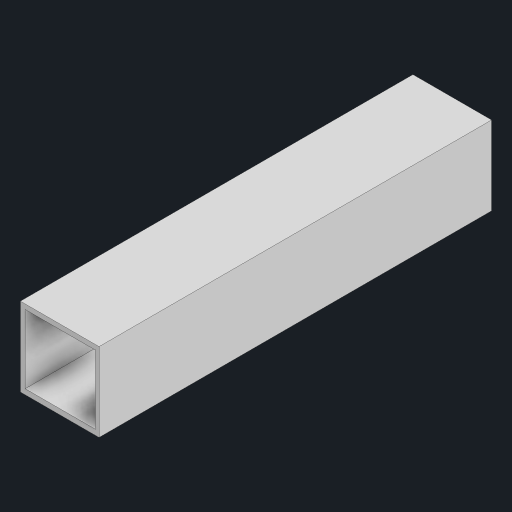
# Autodesk Inventor part: support
Saved by Autodesk Inventor 2024 (Build 280153000, 153)
## iProperties
Created: 2023-11-07
Part Number: support
Material: Generic
Document SubType Name: Modeling
Designer: 91840
Density: 1 g/cm^3
Appearance: Default
Author: 91840
Autodesk Inventor part; units mm, degrees
ref_plane "YZ Plane" through (0, 0, 0) normal (1, 0, 0) x (0, 1, 0)
ref_plane "XZ Plane" through (0, 0, 0) normal (0, 1, 0) x (-1, 0, 0)
ref_plane "XY Plane" through (0, 0, 0) normal (0, 0, 1) x (1, 0, 0)
sketch "Sketch1" plane through (0, 0, 0) normal (0, 0, 1) x (1, 0, 0)
  line L0 (-8, 7) -> (41.3, 7)
  line L1 (41.3, 7) -> (41.3, -42.3)
  line L2 (41.3, -42.3) -> (-8, -42.3)
  line L3 (-8, -42.3) -> (-8, 7)
  point P0 (0, 0)
  dimension "d0" = 49.3
  dimension "d1" = 49.3
  constraints: 8 end point, 2 parallel, 1 horizontal, 1 perpendicular
  measures "d0" distance of L1.end L2.end
  measures "d1" distance of L0.end L1.end
extrude "Extrusion1" add sketch "Sketch1" along normal blind 246
sketch "Sketch2" plane through (0, 0, 246) normal (0, 0, 1) x (1, 0, 0)
  line L0 (-5, 4) -> (39, 4)
  line L1 (39, 4) -> (39, -39)
  line L2 (39, -39) -> (-5, -39)
  line L3 (-5, -39) -> (-5, 4)
  point P0 (0, 0)
  constraints: 8 end point, 2 parallel, 1 horizontal, 1 perpendicular
extrude "Extrusion2" cut sketch "Sketch2" against normal through all
body "Solid1"
